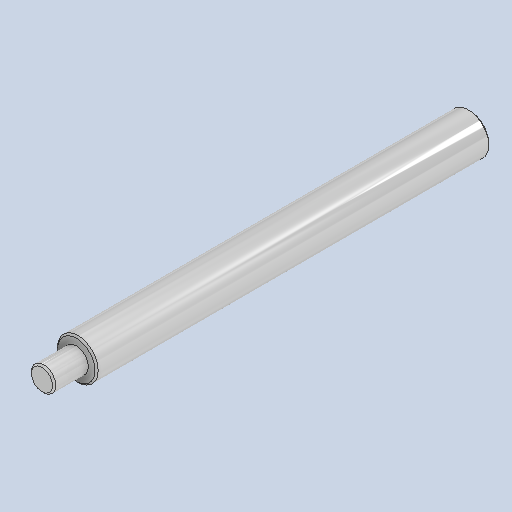
# Autodesk Inventor part: SensorKopf_Encoder_Welle
Saved by Autodesk Inventor 2024 (Build 280153000, 153)
## iProperties
Created: 2023-07-31
Part Number: SensorKopf_Encoder_Welle
Material: Aluminum 6061-AHC
Document SubType Name: Modeling
Designer: aewalder
Mass: 2.34704 g
Surface Area: 7.46214 cm^2
Volume: 0.869272 cm^3
Density: 2.7 g/cm^3
Appearance: Aluminum - Dark
Author: aewalder
Autodesk Inventor part; units mm, degrees
ref_plane "YZ Plane" through (0, 0, 0) normal (1, 0, 0) x (0, 1, 0)
ref_plane "XZ Plane" through (0, 0, 0) normal (0, 1, 0) x (-1, 0, 0)
ref_plane "XY Plane" through (0, 0, 0) normal (0, 0, 1) x (1, 0, 0)
sketch "Sketch1" plane through (0, 0, 0) normal (0, 0, 1) x (1, 0, 0)
  circle A0 centre (0, 0) radius 2.5
  dimension "d0" = 5
  constraints: 1 centre point, 1 coincident
  measures "d0" diameter of A0
extrude "Extrusion1" add sketch "Sketch1" along normal blind 52.5
sketch "Sketch2" plane through (0, 0, 52.5) normal (0, 0, 1) x (1, 0, 0)
  circle A0 centre (0, 0) radius 2.5 projected
  circle A1 centre (0, 0) radius 1.5
  dimension "d3" = 3
  constraints: 1 centre point, 1 coincident
  measures "d3" diameter of A1
extrude "Extrusion2" cut sketch "Sketch2" against normal blind 4.2
chamfer "Chamfer1" distance 0.2 angle 45 3 edges at (-1.5, 0, 52.5) (-2.5, 0, 48.3) (-2.5, 0, 0)
body "Solid1"
